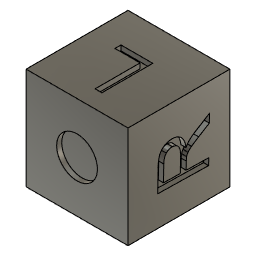
LCR cube v1 (Autodesk Fusion 360 design; units mm, degrees)
Autodesk Fusion 360 part; units mm, degrees
sketch "Sketch1" plane through (0, 0, 0) normal (0, 0, 1) x (1, 0, 0) in component "Tets"
  line L0 (10, -10) -> (-10, -10)
  line L1 (-10, -10) -> (-10, 10)
  line L2 (-10, 10) -> (10, 10)
  line L3 (10, 10) -> (10, -10)
  line L4 (10, -10) -> (-10, 10) construction
  line L5 (-10, -10) -> (10, 10) construction
  constraint horizontal L0
  constraint perpendicular L0 L1
  constraint parallel L0 L2
  constraint parallel L1 L3
  constraint coincident L4 origin
  constraint coincident L5 origin
extrude "Extrude1" add sketch "Sketch1" along normal blind 20 in component "Tets"
sketch "Sketch2" plane through (0, 0, 20) normal (0, 0, 1) x (-1, 0, 0) in component "Tets"
  line L0 (-10, -10) -> (10, -10)
  line L1 (10, -10) -> (10, 10)
  line L2 (10, 10) -> (-10, 10)
  line L3 (-10, 10) -> (-10, -10)
  line L4 (-1.4417, -13.4233) -> (18.5583, -13.4233) construction
  line L5 (18.5583, -13.4233) -> (18.5583, 6.5767) construction
  line L6 (18.5583, 6.5767) -> (-1.4417, 6.5767) construction
  line L7 (-1.4417, 6.5767) -> (-1.4417, -13.4233) construction
  dimension "d3" = 10
  text T0 "L" font "Arial" height 10 align left top in box 20 x 20 at (-1.4417, -13.4233) x (1, 0) y (0, 1) spacing 1 kerned
extrude "Extrude2" cut sketch "Sketch2" against normal blind 1 text T0 in component "Tets"
sketch "Sketch4" plane through (0, 0, 0) normal (0, 0, -1) x (1, 0, 0) in component "Tets"
  line L0 (-10, -10) -> (10, -10)
  line L1 (10, -10) -> (10, 10)
  line L2 (10, 10) -> (-10, 10)
  line L3 (-10, 10) -> (-10, -10)
  line L4 (2.5778, 6.312) -> (-8.4222, 6.312) construction
  line L5 (-8.4222, 6.312) -> (-8.4222, -3.688) construction
  line L6 (-8.4222, -3.688) -> (2.5778, -3.688) construction
  line L7 (2.5778, -3.688) -> (2.5778, 6.312) construction
  dimension "d9" = 10
  text T0 "c" font "Arial" height 10 align left top in box 11 x 10 at (2.5778, 6.312) x (-1, 0) y (0, -1) spacing 1 kerned
extrude "Extrude4" cut sketch "Sketch4" against normal blind 1 text T0 in component "Tets"
sketch "Sketch5" plane through (10, 0, 0) normal (1, 0, 0) x (0, 1, 0) in component "Tets"
  line L0 (-10, 0) -> (10, 0)
  line L1 (10, 0) -> (10, 20)
  line L2 (10, 20) -> (-10, 20)
  line L3 (-10, 20) -> (-10, 0)
  line L4 (0.7139, 4.7063) -> (0.8412, 11.1444) construction
  line L5 (0.8412, 11.1444) -> (-6.7139, 11.2937) construction
  line L6 (-6.7139, 11.2937) -> (-6.8412, 4.8556) construction
  line L7 (-6.8412, 4.8556) -> (0.7139, 4.7063) construction
  dimension "d12" = 10
  text T0 "R" font "Arial" height 10 align left top in box 6.4393 x 7.5566 at (0.7139, 4.7063) x (0.019764, 0.999805) y (-0.999805, 0.019764) spacing 1 kerned
extrude "Extrude5" cut sketch "Sketch5" against normal blind 1 text T0 in component "Tets"
sketch "Sketch6" plane through (0, 10, 0) normal (0, 1, 0) x (-1, 0, 0) in component "Tets"
  line L0 (-10, 0) -> (10, 0)
  line L1 (10, 0) -> (10, 20)
  line L2 (10, 20) -> (-10, 20)
  line L3 (-10, 20) -> (-10, 0)
  circle A0 centre (0, 10) radius 4
  dimension "d15" = 8
  measures "d15" diameter of A0
extrude "Extrude6" cut sketch "Sketch6" against normal blind 1 contours A0 in component "Tets"
sketch "Sketch7" plane through (-10, 0, 0) normal (-1, 0, 0) x (0, -1, 0) in component "Tets"
  line L0 (-10, 0) -> (10, 0)
  line L1 (10, 0) -> (10, 20)
  line L2 (10, 20) -> (-10, 20)
  line L3 (-10, 20) -> (-10, 0)
  circle A0 centre (0, 10) radius 4
  dimension "d18" = 8
  measures "d18" diameter of A0
extrude "Extrude7" cut sketch "Sketch7" against normal blind 1 contours A0 in component "Tets"
sketch "Sketch8" plane through (0, -10, 0) normal (0, -1, 0) x (1, 0, 0) in component "Tets"
  line L0 (-10, 0) -> (10, 0)
  line L1 (10, 0) -> (10, 20)
  line L2 (10, 20) -> (-10, 20)
  line L3 (-10, 20) -> (-10, 0)
  circle A0 centre (0, 10) radius 4
  dimension "d21" = 8
  measures "d21" diameter of A0
extrude "Extrude8" cut sketch "Sketch8" against normal blind 1 contours A0 in component "Tets"
component "Tets" placed x (1, 0, 0) y (0, 1, 0) z (0, 0, 1) at (0, 0, 0)
